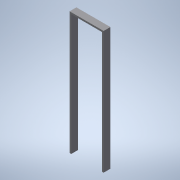
# Autodesk Inventor part: arm1
Saved by Autodesk Inventor 2020 (Build 240168000, 168)
## iProperties
Created: 2021-06-01
Part Number: arm1
Material: 一般
Document SubType Name: Modeling
Designer: yossy
Density: 1 g/cm^3
Appearance: 既定
Author: yossy
Autodesk Inventor part; units mm, degrees
ref_plane "YZ Plane" through (0, 0, 0) normal (1, 0, 0) x (0, 1, 0)
ref_plane "XZ Plane" through (0, 0, 0) normal (0, 1, 0) x (-1, 0, 0)
sketch "スケッチ1" plane through (0, 0, 0) normal (0, 0, 1) x (1, 0, 0)
  line L0 (0, 0) -> (-100, 0)
  line L1 (-100, 0) -> (-100, -360)
  line L2 (-100, -360) -> (0, -360)
  line L3 (0, -360) -> (0, 0)
  dimension "d0" = 100
  dimension "d1" = 360
  constraints: 8 end point, 2 parallel, 1 horizontal, 1 perpendicular
  measures "d0" distance of L2.end L1.end
  measures "d1" distance of L1.end L0.end
ref_plane "作業平面1" through (-6, -360, -20) normal (0, 0, -1) x (0, 1, 0)
extrude "押し出し1" add sketch "スケッチ1" against normal up to surface (20 mm away)
sketch "スケッチ3" plane through (0, 0, 0) normal (0, 0, 1) x (1, 0, 0)
  line L0 (0, -360) -> (0, 0) projected
  line L1 (0, 0) -> (-100, 0) projected
  line L2 (-100, 0) -> (-100, -360) projected
  line L3 (-100, -360) -> (0, -360) projected
  line L4 (-5, -5) -> (-95, -5)
  line L5 (-95, -5) -> (-95, -360)
  line L6 (-95, -360) -> (-5, -360)
  line L7 (-5, -360) -> (-5, -5)
  point P0 (-5, -360)
  dimension "d4" = 5
  dimension "d5" = 5
  dimension "d6" = 5
  dimension "d7" = 0
  constraints: 8 end point, 2 parallel, 1 horizontal, 1 perpendicular
  measures "d4" distance between parallel lines of L1 L4
  measures "d5" distance between parallel lines of L0 L7
  measures "d6" distance between parallel lines of L2 L5
  measures "d7" distance between parallel lines of L3 L6
extrude "押し出し2" cut sketch "スケッチ3" against normal up to surface (20 mm away) contours L3 L5 L4 L7
